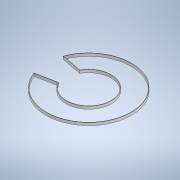
# Autodesk Inventor part: Level 3 Edge Banding
Saved by Autodesk Inventor 2021 (Build 250183000, 183)
## iProperties
Created: 2020-10-10
Part Number: Level 3 Edge Banding
Material: Generic
Document SubType Name: Modeling
Designer: Daniel Wikman
Density: 1 g/cm^3
Appearance: Default
Author: Daniel Wikman
Autodesk Inventor part; units mm, degrees
ref_plane "YZ Plane" through (0, 0, 0) normal (1, 0, 0) x (0, 1, 0)
ref_plane "XZ Plane" through (0, 0, 0) normal (0, 1, 0) x (-1, 0, 0)
ref_plane "XY Plane" through (0, 0, 0) normal (0, 0, 1) x (1, 0, 0)
sketch "Sketch1" plane through (0, 0, 0) normal (0, 1, 0) x (-1, 0, 0)
  arc A0 (164.6416, -27.5) -> (351.8594, -257.6833) centre (416.6605, -13.75) ccw
  arc A1 (351.8594, -257.6833) -> (637.4975, -135.9533) centre (416.6605, -13.75) ccw
  arc A2 (637.4975, 108.4533) -> (325.7053, 221.6853) centre (416.6605, -13.75) ccw
  arc A3 (325.7053, 221.6853) -> (164.6416, -27.5) centre (416.6605, -13.75) ccw
  line L0 (859.1908, 151.5461) -> (637.4975, 108.4533)
  line L1 (637.4975, -135.9533) -> (859.1908, -179.0461)
  arc A4 (283.8217, -467.0818) -> (859.1908, -179.0461) centre (416.6605, -13.75) ccw
  arc A5 (637.4975, 108.4533) -> (637.4975, -135.9533) centre (416.6605, -13.75) ccw
  arc A6 (859.1908, 151.5461) -> (859.1908, -179.0461) centre (416.6605, -13.75) ccw
  arc A7 (864.5675, 148.5163) -> (864.5675, -176.0163) centre (416.6605, -13.75) ccw
  arc A8 (635.3883, 103.9684) -> (635.3883, -131.4684) centre (416.6605, -13.75) ccw
  line L2 (635.3883, -131.4684) -> (864.5675, -176.0163)
  line L3 (635.3883, 103.9684) -> (864.5675, 148.5163)
  point P0 (0, 0)
  point P1 (283.8217, -467.0818)
  dimension "d0" = 4
  dimension "d1" = 4
  dimension "d2" = 4
  dimension "d3" = 4
  constraints: 20 point on circle, 9 centre point, 8 end point, 4 coincident, 4 point on line, 2 parallel
  measures "d0" radial gap between concentric circles of A1 A8
  measures "d1" radial gap between concentric circles of A6 A7
  measures "d2" distance between parallel lines of L1 L2
  measures "d3" distance between parallel lines of L0 L3
extrude "Extrusion1" add sketch "Sketch1" along normal blind 30
body "Solid1"
